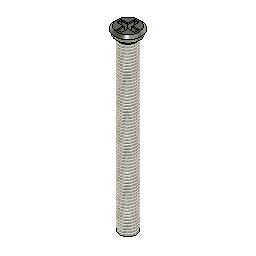
Bolt-M5 (Autodesk Fusion 360 design; units mm, degrees)
part number: 2026-04-18-16-33-04-070
Autodesk Fusion 360 part; units mm, degrees
sketch "Sketch1" plane through (0, 0, 0) normal (0, 0, 1) x (1, 0, 0)
  circle A0 centre (0, 0) radius 4
  dimension "d1" = 8
  constraint coincident A0.centre origin
  measures "d1" diameter of A0
extrude "Extrude1" add sketch "Sketch1" along normal blind 3
sketch "Sketch2" plane through (0, 0, 0) normal (0, 0, -1) x (1, 0, 0)
  circle A0 centre (0, 0) radius 4
  circle A1 centre (0, 0) radius 2.5
  dimension "d4" = 5
  constraint coincident A0.centre A1.centre
  measures "d4" diameter of A1
extrude "Extrude2" add sketch "Sketch2" along normal blind 50 contours A1
sketch "Sketch3" plane through (0, 0, 3) normal (0, 0, 1) x (-1, 0, 0)
  circle A0 centre (0, 0) radius 4
  line L0 (0.5, 2.5) -> (-0.5, 2.5)
  line L1 (-0.5, 2.5) -> (-0.5, -2.5)
  line L2 (-0.5, -2.5) -> (0.5, -2.5)
  line L3 (0.5, -2.5) -> (0.5, 2.5)
  line L4 (0.5, 2.5) -> (-0.5, -2.5) construction
  line L5 (-0.5, 2.5) -> (0.5, -2.5) construction
  line L6 (2.5, 0.5) -> (-2.5, 0.5)
  line L7 (-2.5, 0.5) -> (-2.5, -0.5)
  line L8 (-2.5, -0.5) -> (2.5, -0.5)
  line L9 (2.5, -0.5) -> (2.5, 0.5)
  line L10 (2.5, 0.5) -> (-2.5, -0.5) construction
  line L11 (-2.5, 0.5) -> (2.5, -0.5) construction
  dimension "d9" = 1
  dimension "d10" = 5
  dimension "d11" = 5
  dimension "d12" = 1
  constraint horizontal L0
  constraint perpendicular L0 L1
  constraint parallel L0 L2
  constraint parallel L1 L3
  constraint coincident L4 A0.centre
  constraint coincident L5 A0.centre
  constraint coincident A0.centre origin
  constraint horizontal L6
  constraint perpendicular L6 L7
  constraint parallel L6 L8
  constraint parallel L7 L9
  constraint coincident L10 A0.centre
  constraint coincident L11 A0.centre
  measures "d9" distance of L1.end L2.end
  measures "d10" distance of L0.end L1.end
  measures "d11" distance of L7.end L8.end
  measures "d12" distance of L6.end L7.end
extrude "Extrude3" cut sketch "Sketch3" against normal blind 2.5 contours L0 L1 L3 L6 | L3 L6 L8 L9 | L1 L3 L6 L8 | L1 L6 L7 L8 | L1 L2 L3 L8
thread "Thread2" "ISO Metric profile 5.0 M5x0.8 M5x0.8 6g" major diameter 4.901 minor diameter 3.9895 pitch 0.8 angle 60 resizes the face on face at (2.4876, 0.2489, -16.6667)
chamfer "Chamfer1" distance 1.5 angle 45 1 edges at (-3.7293, -1.4465, 0)
chamfer "Chamfer2" distance 0.75 angle 45 1 faces at (3.995, 0.1994, 2)
chamfer "Chamfer3" distance 0.2 angle 45 12 edges at (-0.5, 1.5, 3) (-1.5, 0.5, 3) (-2.5, 0, 3) (-1.5, -0.5, 3) (-0.5, -1.5, 3) (0, -2.5, 3) (0.5, -1.5, 3) (1.5, 0.5, 3) (2.5, 0, 3) (1.5, -0.5, 3) (0.5, 1.5, 3) (0, 2.5, 3)
